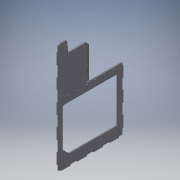
# Autodesk Inventor part: TrayPanelA
Saved by Autodesk Inventor 2017 (Build 210142000, 142)
## iProperties
Created: 2019-06-22
Part Number: TrayPanelA
Material: Generic
Document SubType Name: Modeling
Designer: DDeGo
Density: 1 g/cm^3
Appearance: Default
Author: DDeGo
Autodesk Inventor part; units mm, degrees
ref_plane "YZ Plane" through (0, 0, 0) normal (1, 0, 0) x (0, 1, 0)
ref_plane "XZ Plane" through (0, 0, 0) normal (0, 1, 0) x (-1, 0, 0)
ref_plane "XY Plane" through (0, 0, 0) normal (0, 0, 1) x (1, 0, 0)
sketch "Sketch1" plane through (0, 0, 0) normal (1, 0, 0) x (0, 1, 0)
  line L0 (163, 146.94) -> (163, 32)
  line L1 (15, 151.94) -> (158, 151.94)
  circle A0 centre (8, 187.94) radius 2
  circle A1 centre (69.72, 264.54) radius 2
  circle A2 centre (69.72, 187.94) radius 2
  circle A3 centre (8, 264.54) radius 2
  line L2 (83, 270.54) -> (20, 300) construction
  line L3 (0, 0) -> (0, 300)
  line L4 (175, 0) -> (0, 0)
  line L5 (175, 0) -> (175, 172)
  line L6 (83, 172) -> (175, 172)
  line L7 (83, 172) -> (83, 270.54)
  circle A4 centre (10.52, 166.94) radius 1.2
  circle A5 centre (168, 12) radius 1.2
  circle A6 centre (168, 166.94) radius 1.2
  circle A7 centre (10.52, 34.86) radius 1.2
  line L8 (10.52, 166.94) -> (168, 166.94) construction
  line L9 (168, 166.94) -> (168, 12) construction
  line L10 (168, 12) -> (10.52, 12) construction
  line L11 (10.52, 12) -> (10.52, 34.86) construction
  line L12 (10.52, 34.86) -> (10.52, 166.94) construction
  line L13 (20, 300) -> (0, 300)
  line L14 (8, 264.54) -> (69.72, 264.54) construction
  line L15 (69.72, 264.54) -> (69.72, 187.94) construction
  line L16 (69.72, 187.94) -> (8, 187.94) construction
  line L17 (8, 187.94) -> (8, 264.54) construction
  line L18 (166.65, 0) -> (141.5, 0)
  line L19 (141.5, 0) -> (141.5, -3)
  line L20 (141.5, -3) -> (166.65, -3)
  line L21 (166.65, -3) -> (166.65, 0)
  line L22 (121.65, 0) -> (96.5, 0)
  line L23 (96.5, 0) -> (96.5, -3)
  line L24 (96.5, -3) -> (121.65, -3)
  line L25 (121.65, -3) -> (121.65, 0)
  line L26 (76.65, 0) -> (51.5, 0)
  line L27 (51.5, 0) -> (51.5, -3)
  line L28 (51.5, -3) -> (76.65, -3)
  line L29 (76.65, -3) -> (76.65, 0)
  line L30 (31.65, 0) -> (6.5, 0)
  line L31 (6.5, 0) -> (6.5, -3)
  line L32 (6.5, -3) -> (31.65, -3)
  line L33 (31.65, -3) -> (31.65, 0)
  line L34 (0, 285.15) -> (-3, 285.15)
  line L35 (-3, 285.15) -> (-3, 255)
  line L36 (-3, 255) -> (0, 255)
  line L37 (0, 255) -> (0, 285.15)
  line L38 (0, 225.15) -> (-3, 225.15)
  line L39 (-3, 225.15) -> (-3, 195)
  line L40 (-3, 195) -> (0, 195)
  line L41 (0, 195) -> (0, 225.15)
  line L42 (0, 165.15) -> (-3, 165.15)
  line L43 (-3, 165.15) -> (-3, 135)
  line L44 (-3, 135) -> (0, 135)
  line L45 (0, 135) -> (0, 165.15)
  line L46 (0, 105.15) -> (-3, 105.15)
  line L47 (-3, 105.15) -> (-3, 75)
  line L48 (-3, 75) -> (0, 75)
  line L49 (0, 75) -> (0, 105.15)
  line L50 (0, 45.15) -> (-3, 45.15)
  line L51 (-3, 45.15) -> (-3, 15)
  line L52 (-3, 15) -> (0, 15)
  line L53 (0, 15) -> (0, 45.15)
  line L54 (175, 165.15) -> (178, 165.15)
  line L55 (178, 165.15) -> (178, 135)
  line L56 (178, 135) -> (175, 135)
  line L57 (175, 135) -> (175, 165.15)
  line L58 (175, 105.15) -> (178, 105.15)
  line L59 (178, 105.15) -> (178, 75)
  line L60 (178, 75) -> (175, 75)
  line L61 (175, 75) -> (175, 105.15)
  line L62 (175, 45.15) -> (178, 45.15)
  line L63 (178, 45.15) -> (178, 15)
  line L64 (178, 15) -> (175, 15)
  line L65 (175, 15) -> (175, 45.15)
  line L66 (83, 270.54) -> (25, 270.54)
  line L67 (20, 300) -> (5, 300)
  line L68 (5, 300) -> (5, 302.5)
  line L69 (5, 302.5) -> (20, 302.5)
  line L70 (20, 302.5) -> (20, 300)
  line L71 (11.4645, 43.3955) -> (26.3955, 28.4645)
  line L72 (10, 46.9311) -> (10, 146.94)
  line L73 (158, 27) -> (29.9311, 27)
  arc A8 (163, 146.94) -> (158, 151.94) centre (158, 146.94) ccw
  arc A9 (158, 27) -> (163, 32) centre (158, 32) ccw
  arc A10 (15, 151.94) -> (10, 146.94) centre (15, 146.94) ccw
  arc A11 (10, 46.9311) -> (11.4645, 43.3955) centre (15, 46.9311) ccw
  arc A12 (26.3955, 28.4645) -> (29.9311, 27) centre (29.9311, 32) ccw
  line L74 (20, 300) -> (22, 300)
  line L75 (22, 300) -> (25, 270.54)
  point P0 (163, 151.94)
  point P1 (163, 27)
  point P2 (10, 151.94)
  point P3 (10, 44.86)
  dimension "d48" = 10
  dimension "d2" = 175
  dimension "d3" = 172
  dimension "d4" = 157.48
  dimension "d5" = 154.94
  dimension "d6" = 7
  dimension "d7" = 12
  dimension "d8" = 83
  dimension "d9" = 20
  dimension "d16" = 61.72
  dimension "d17" = 76.6
  dimension "d18" = 21
  dimension "d19" = 8
  dimension "d20" = 2.4
  dimension "d21" = 22.86
  dimension "d22" = 4
  dimension "d23" = 3
  dimension "d24" = 25.15
  dimension "d25" = 45
  dimension "d26" = 45
  dimension "d27" = 45
  dimension "d28" = 6.5
  dimension "d29" = 30.15
  dimension "d30" = 60
  dimension "d31" = 60
  dimension "d32" = 60
  dimension "d33" = 60
  dimension "d34" = 15
  dimension "d35" = 3
  dimension "d36" = 3
  dimension "d37" = 30.15
  dimension "d38" = 15
  dimension "d39" = 60
  dimension "d40" = 60
  dimension "d50" = 5
  dimension "d51" = 2.5
  dimension "d52" = 15
  dimension "d53" = 300
  dimension "d54" = 15
  dimension "d55" = 10
  dimension "d56" = 10
  dimension "d57" = 45
  dimension "d59" = 5
  dimension "d60" = 2
  dimension "d62" = 6
  dimension "d63" = 5
  dimension "d64" = 15
  constraints: 152 end point, 29 point on line, 27 parallel, 19 perpendicular, 17 horizontal, 15 equal length, 13 centre point, 10 equal radius, 10 point on circle, 10 tangent, 1 coincident, 1 collinear, 1 vertical
  measures "d2" distance of L4.start L3.start
  measures "d3" distance between parallel lines of L4 L6
  measures "d4" horizontal distance of L11.end L9.end
  measures "d5" distance of L8.end L9.end
  measures "d6" distance between parallel lines of L5 L9
  measures "d7" distance between parallel lines of L4 L10
  measures "d8" distance between parallel lines of L3 L7
  measures "d9" distance of L2.end L3.end
  measures "d16" distance between parallel lines of L15 L17
  measures "d17" distance between parallel lines of L16 L14
  measures "d18" distance between parallel lines of L16 L8
  measures "d19" distance between parallel lines of L3 L17
  measures "d20" diameter of A4
  measures "d21" vertical distance of L9.end L11.end
  measures "d22" diameter of A3
  measures "d23" distance between parallel lines of L4 L20
  measures "d24" distance of L19.end L20.end
  measures "d25" distance between parallel lines of L27 L31
  measures "d26" distance between parallel lines of L27 L23
  measures "d27" distance between parallel lines of L19 L23
  measures "d28" distance between parallel lines of L3 L31
  measures "d29" distance of L34.end L35.end
  measures "d30" distance between parallel lines of L38 L34
  measures "d31" distance between parallel lines of L42 L38
  measures "d32" distance between parallel lines of L46 L42
  measures "d33" distance between parallel lines of L50 L46
  measures "d34" distance between parallel lines of L4 L52
  measures "d35" distance of L50.start L50.end
  measures "d36" distance of L54.start L54.end
  measures "d37" distance of L62.end L63.end
  measures "d38" distance from line of L4.start L64
  measures "d39" distance of L59.end L63.end
  measures "d40" distance of L55.end L59.end
  measures "d50" horizontal distance of L2.end L66.end
  measures "d51" distance of L67.end L68.end
  measures "d52" distance of L68.end L69.end
  measures "d53" distance between parallel lines of L4 L67
  measures "d54" distance between parallel lines of L10 L73
  measures "d55" distance between parallel lines of L3 L72
  measures "d56" vertical distance of L11.end point (10, 44.86)
  measures "d57" angle of L72 L71
  measures "d59" radius of A8
  measures "d60" distance of L2.end L74.end
  measures "d62" distance between parallel lines of L66 L14
  measures "d63" distance between parallel lines of L0 L9
  measures "d64" distance between parallel lines of L1 L8
extrude "Extrusion1" add sketch "Sketch1" along normal blind 2.75
sketch "Sketch2" plane through (2.75, 0, 0) normal (1, 0, 0) x (0, 0, -1)
  line L0 (-172, 175) -> (-172, 83) projected
  line L1 (-172, 83) -> (-176.3, 83)
  line L2 (-176.3, 83) -> (-176.3, 76)
  line L3 (-176.3, 76) -> (-172, 76)
  line L4 (-172, 76) -> (-172, 83)
  line L5 (-172, 88.5) -> (-167.8, 88.5)
  line L6 (-167.8, 91.5) -> (-172, 91.5)
  line L7 (-172, 91.5) -> (-172, 88.5)
  line L8 (-167.8, 92.75) -> (-165.3, 92.75)
  line L9 (-165.3, 92.75) -> (-165.3, 87.25)
  line L10 (-165.3, 87.25) -> (-167.8, 87.25)
  line L11 (-167.8, 87.25) -> (-167.8, 88.5)
  line L12 (-167.8, 91.5) -> (-167.8, 92.75)
  line L13 (-172, 83) -> (-270.54, 83) projected
  point P0 (0, 0)
  point P1 (-172, 90)
  dimension "d41" = 5.5
  dimension "d42" = 2.5
  dimension "d44" = 4.3
  dimension "d45" = 7
  dimension "d46" = 7
  dimension "d47" = 3
  dimension "d61" = 11
  constraints: 24 end point, 6 parallel, 3 horizontal, 2 collinear, 2 perpendicular, 2 point on line, 1 midpoint
  measures "d41" distance between parallel lines of L8 L10
  measures "d42" distance of L9.end L10.end
  measures "d44" distance between parallel lines of L4 L2
  measures "d45" distance of L3.end L0.end
  measures "d46" distance from line of L13 point (-172, 90)
  measures "d47" distance between parallel lines of L6 L5
  measures "d61" distance between parallel lines of L9 L2
extrude "Extrusion2" cut sketch "Sketch2" against normal blind 10
sketch "Sketch3" plane through (0, 0, 0) normal (-1, 0, 0) x (0, 0, 1)
  line L0 (270.54, 75.15) -> (257.3, 75.15)
  line L1 (257.3, 75.15) -> (257.3, 77.9)
  line L2 (257.3, 77.9) -> (270.54, 77.9)
  line L3 (270.54, 77.9) -> (270.54, 75.15)
  line L4 (176.3, 83) -> (270.54, 83) projected
  line L5 (176.3, 83) -> (176.3, 76) projected
  line L6 (270.54, 83) -> (270.54, 25) projected
  point P0 (0, 0)
  dimension "d65" = 2.75
  dimension "d67" = 5.1
  dimension "d68" = 81
  constraints: 8 end point, 2 parallel, 1 horizontal, 1 perpendicular, 1 point on line
  measures "d65" distance between parallel lines of L0 L2
  measures "d67" distance between parallel lines of L4 L2
  measures "d68" distance between parallel lines of L5 L1
extrude "Extrusion3" cut sketch "Sketch3" against normal blind 10
sketch "Sketch4" plane through (2.75, 0, 0) normal (1, 0, 0) x (0, 0, -1)
  line L0 (-242.3, 78.5) -> (-252.3, 78.5)
  line L1 (-252.3, 78.5) -> (-252.3, 80.5)
  line L2 (-252.3, 80.5) -> (-242.3, 80.5)
  line L3 (-242.3, 80.5) -> (-242.3, 78.5)
  line L4 (-176.3, 83) -> (-270.54, 83) projected
  line L5 (-257.3, 77.9) -> (-257.3, 75.15) projected
  line L6 (-219.3, 78.5) -> (-229.3, 78.5)
  line L7 (-229.3, 78.5) -> (-229.3, 80.5)
  line L8 (-229.3, 80.5) -> (-219.3, 80.5)
  line L9 (-219.3, 80.5) -> (-219.3, 78.5)
  line L10 (-196.3, 78.5) -> (-206.3, 78.5)
  line L11 (-206.3, 78.5) -> (-206.3, 80.5)
  line L12 (-206.3, 80.5) -> (-196.3, 80.5)
  line L13 (-196.3, 80.5) -> (-196.3, 78.5)
  line L14 (-167.5, 158) -> (-169.5, 158)
  line L15 (-169.5, 158) -> (-169.5, 148)
  line L16 (-169.5, 148) -> (-167.5, 148)
  line L17 (-167.5, 148) -> (-167.5, 158)
  line L18 (-172, 175) -> (-172, 91.5) projected
  circle A0 centre (-166.94, 168) radius 1.2 projected
  line L19 (-169.5, 123) -> (-167.5, 123)
  line L20 (-169.5, 133) -> (-169.5, 123)
  line L21 (-167.5, 123) -> (-167.5, 133)
  line L22 (-167.5, 133) -> (-169.5, 133)
  line L23 (-169.5, 98) -> (-167.5, 98)
  line L24 (-169.5, 108) -> (-169.5, 98)
  line L25 (-167.5, 98) -> (-167.5, 108)
  line L26 (-167.5, 108) -> (-169.5, 108)
  line L27 (-169.5, 73) -> (-167.5, 73)
  line L28 (-169.5, 83) -> (-169.5, 73)
  line L29 (-167.5, 73) -> (-167.5, 83)
  line L30 (-167.5, 83) -> (-169.5, 83)
  line L31 (-169.5, 48) -> (-167.5, 48)
  line L32 (-169.5, 58) -> (-169.5, 48)
  line L33 (-167.5, 48) -> (-167.5, 58)
  line L34 (-167.5, 58) -> (-169.5, 58)
  line L35 (-169.5, 23) -> (-167.5, 23)
  line L36 (-169.5, 33) -> (-169.5, 23)
  line L37 (-167.5, 23) -> (-167.5, 33)
  line L38 (-167.5, 33) -> (-169.5, 33)
  point P0 (0, 0)
  dimension "d71" = 10
  dimension "d72" = 2
  dimension "d73" = 2.5
  dimension "d74" = 5
  dimension "d77" = 23
  dimension "d82" = 10
  dimension "d83" = 2
  dimension "d84" = 2.5
  dimension "d85" = 10
  dimension "d88" = 25
  constraints: 72 end point, 4 parallel, 3 horizontal, 2 perpendicular, 1 vertical, 56 other
  measures "d71" distance of L0.start L0.end
  measures "d72" distance of L2.end L0.start
  measures "d73" distance between parallel lines of L4 L2
  measures "d74" distance from line of L1.end L5
  measures "d77" distance of L0.start L6.start
  measures "d82" distance of L14.end L15.end
  measures "d83" distance of L15.end L16.end
  measures "d84" distance between parallel lines of L18 L15
  measures "d85" distance from line of A0.centre L14
  measures "d88" distance of L15.end L19.start
extrude "Extrusion4" cut sketch "Sketch4" against normal through all
sketch "Sketch5" plane through (2.75, 0, 0) normal (1, 0, 0) x (0, 0, -1)
  line L0 (-257.3, 77.9) -> (-270.54, 77.9) projected
  line L1 (-267.54, 77.9) -> (-262.44, 83)
  line L2 (-270.54, 83) -> (-270.54, 77.9) projected
  line L3 (-262.44, 83) -> (-270.54, 83)
  line L4 (-270.54, 83) -> (-270.54, 77.9)
  line L5 (-270.54, 77.9) -> (-267.54, 77.9)
  point P0 (0, 0)
  dimension "d95" = 3
  dimension "d96" = 45
  constraints: 8 end point, 3 perpendicular, 1 point on line
  measures "d95" distance of L0.end L1.start
  measures "d96" angle of L3 L1
extrude "Extrusion5" cut sketch "Sketch5" against normal blind 10
equation "\"d26\" = d25"
equation "\"d27\" = d25"
equation "\"d31\" = d30"
equation "\"d32\" = d30"
equation "\"d33\" = d30"
equation "\"d40\" = d39"
body "Solid1"
